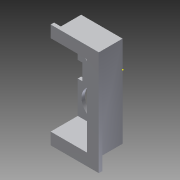
# Autodesk Inventor part: Sonar_Bracket
Saved by Autodesk Inventor 2015 (Build 190159000, 159)
## iProperties
Created: 2017-03-19
Part Number: Sonar_Bracket
Material: ABS Plastic
Document SubType Name: Modeling
Designer: ks2101
Density: 1.06 g/cm^3
Appearance: Smooth - White
Author: ks2101
Autodesk Inventor part; units mm, degrees
ref_plane "YZ Plane" through (0, 0, 0) normal (1, 0, 0) x (0, 1, 0)
ref_plane "XZ Plane" through (0, 0, 0) normal (0, 1, 0) x (-1, 0, 0)
ref_plane "XY Plane" through (0, 0, 0) normal (0, 0, 1) x (1, 0, 0)
sketch "Sketch1" plane through (0, 0, 0) normal (0, 0, 1) x (1, 0, 0)
  line L0 (-2.6984, 15.8681) -> (21.7216, 15.8681)
  line L1 (21.7216, 15.8681) -> (21.7216, -37.8319)
  line L2 (21.7216, -37.8319) -> (-2.6984, -37.8319)
  line L3 (-2.6984, -37.8319) -> (-2.6984, 15.8681)
  point P0 (0, 0)
  dimension "d0" = 53.7
  dimension "d1" = 24.42
  constraints: 8 end point, 2 parallel, 1 horizontal, 1 perpendicular
  measures "d0" distance of L1.end L0.end
  measures "d1" distance of L0.start L0.end
extrude "Extrusion1" add sketch "Sketch1" along normal blind 2
sketch "Sketch2" plane through (0, 0, 2) normal (0, 0, 1) x (1, 0, 0)
  line L0 (-2.6984, -37.8319) -> (21.7216, -37.8319) projected
  line L1 (21.7216, 15.8681) -> (18.7216, 15.8681)
  line L2 (18.7216, 15.8681) -> (18.7216, -37.8319)
  line L3 (18.7216, -37.8319) -> (21.7216, -37.8319)
  line L4 (21.7216, -37.8319) -> (21.7216, 15.8681)
  line L5 (21.7216, -37.8319) -> (21.7216, 15.8681) projected
  line L6 (-2.6984, 15.8681) -> (21.7216, 15.8681)
  line L7 (21.7216, 15.8681) -> (21.7216, 12.8681)
  line L8 (21.7216, 12.8681) -> (-2.6984, 12.8681)
  line L9 (-2.6984, 12.8681) -> (-2.6984, 15.8681)
  line L10 (-2.6984, -37.8319) -> (21.7216, -37.8319)
  line L11 (21.7216, -37.8319) -> (21.7216, -34.8319)
  line L12 (21.7216, -34.8319) -> (-2.6984, -34.8319)
  line L13 (-2.6984, -34.8319) -> (-2.6984, -37.8319)
  point P0 (0, 0)
  dimension "d4" = 3
  dimension "d5" = 3
  dimension "d6" = 3
  constraints: 24 end point, 6 parallel, 3 horizontal, 3 perpendicular, 3 point on line
  measures "d4" distance of L1.start L1.end
  measures "d5" distance of L7.end L6.end
  measures "d6" distance of L0.end L11.end
extrude "Extrusion2" add sketch "Sketch2" along normal blind 16
sketch "Sketch3" plane through (0, 0, 0) normal (0, 0, -1) x (-1, 0, 0)
  point P0 (0, 0)
sketch "Sketch4" plane through (0, 0, 0) normal (0, 0, -1) x (-1, 0, 0)
  circle A0 centre (-8.0116, 2.4017) radius 8.5
  circle A1 centre (-8.0116, -24.3699) radius 8.5
  line L0 (2.6984, -37.8319) -> (2.6984, 15.8681) projected
  line L1 (-21.7216, -37.8319) -> (2.6984, -37.8319) projected
  line L2 (2.6984, 15.8681) -> (-21.7216, 15.8681) projected
  line L3 (-18.7216, 12.8681) -> (-18.7216, -34.8319) projected
  point P0 (0, 0)
  dimension "d9" = 17
  dimension "d10" = 17
  dimension "d11" = 10.71
  dimension "d12" = 10.71
  dimension "d13" = 26.7716
  dimension "d14" = 13.462
  dimension "d15" = 13.4664
  dimension "d45" = 24.42
  dimension "d46" = 21.42
  constraints: 2 centre point
  measures "d9" diameter of A0
  measures "d10" diameter of A1
  measures "d11" distance from line of L0 A0.centre
  measures "d12" distance from line of L0 A1.centre
  measures "d13" distance of A1.centre A0.centre
  measures "d14" distance from line of L1 A1.centre
  measures "d15" distance from line of L2 A0.centre
  measures "d45" distance of L0.end L2.end
  measures "d46" distance between parallel lines of L3 L0
hole "Hole1" at (8.0116, 2.4017, 0) at (8.0116, -24.3699, 0) direction (0, 0, 1) diameter 17 depth 2 tip angle 118
sketch "Sketch5" plane through (0, 0, 2) normal (0, 0, 1) x (1, 0, 0)
  line L0 (-0.1076, -6.2299) -> (-2.6984, -6.2299)
  line L1 (-2.6984, -6.2299) -> (-2.6984, -15.7299)
  line L2 (-2.6984, -15.7299) -> (-0.1076, -15.7299)
  line L3 (-0.1076, -15.7299) -> (-0.1076, -6.2299)
  line L4 (21.7216, 15.8681) -> (-2.6984, 15.8681) projected
  line L5 (-2.6984, -37.8319) -> (21.7216, -37.8319) projected
  line L6 (-2.6984, 12.8681) -> (-2.6984, -34.8319) projected
  point P0 (0, 0)
  dimension "d23" = 9.5
  dimension "d24" = 22.098
  dimension "d25" = 22.102
  dimension "d26" = 2.5908
  dimension "d27" = 0
  dimension "d47" = 2.5908
  constraints: 8 end point, 2 parallel, 1 horizontal, 1 perpendicular
  measures "d23" distance of L0.end L1.end
  measures "d24" distance from line of L0.start L4
  measures "d25" distance between parallel lines of L2 L5
  measures "d26" distance of L1.end L2.end
  measures "d27" distance between parallel lines of L6 L1
  measures "d47" distance between parallel lines of L3 L6
extrude "Extrusion3" cut sketch "Sketch5" against normal blind 10
sketch "Sketch6" plane through (0, 0, 2) normal (0, 0, 1) x (1, 0, 0)
  line L0 (17.7216, -5.7319) -> (13.7216, -5.7319)
  line L1 (13.7216, -5.7319) -> (13.7216, -16.2319)
  line L2 (13.7216, -16.2319) -> (17.7216, -16.2319)
  line L3 (17.7216, -16.2319) -> (17.7216, -5.7319)
  line L4 (21.7216, 15.8681) -> (21.7216, -37.8319) projected
  line L5 (-2.6984, -37.8319) -> (21.7216, -37.8319) projected
  line L6 (21.7216, 15.8681) -> (-2.6984, 15.8681) projected
  point P0 (0, 0)
  dimension "d30" = 4
  dimension "d31" = 10.5
  dimension "d32" = 4
  dimension "d33" = 21.6
  dimension "d34" = 21.6
  constraints: 8 end point, 2 parallel, 1 horizontal, 1 perpendicular
  measures "d30" distance of L0.start L0.end
  measures "d31" distance of L0.end L1.end
  measures "d32" distance between parallel lines of L4 L3
  measures "d33" distance between parallel lines of L5 L2
  measures "d34" distance between parallel lines of L6 L0
extrude "Extrusion4" cut sketch "Sketch6" against normal blind 10
sketch "Sketch7" plane through (-2.6984, 15.8681, 0) normal (0, 1, 0) x (1, 0, 0)
  line L0 (0, -2) -> (0, -18) projected
  line L1 (24.42, -18) -> (0, -18)
  line L2 (0, -18) -> (0, -16)
  line L3 (0, -16) -> (24.42, -16)
  line L4 (24.42, -16) -> (24.42, -18)
  point P0 (2.6984, 0)
  dimension "d37" = 2
  constraints: 8 end point, 2 parallel, 1 horizontal, 1 perpendicular, 1 point on line
  measures "d37" distance of L2.end L0.end
extrude "Extrusion5" add sketch "Sketch7" along normal blind 4
sketch "Sketch8" plane through (21.7216, -37.8319, 0) normal (1, 0, 0) x (0, 0, -1)
  point P0 (0, 37.8319)
sketch "Sketch9" plane through (-2.6984, -37.8319, 0) normal (0, -1, 0) x (1, 0, 0)
  line L0 (24.42, 0) -> (24.42, 18) projected
  line L1 (0, 18) -> (24.42, 18)
  line L2 (24.42, 18) -> (24.42, 16)
  line L3 (24.42, 16) -> (0, 16)
  line L4 (0, 16) -> (0, 18)
  point P0 (2.6984, 0)
  dimension "d40" = 2
  constraints: 8 end point, 2 parallel, 1 horizontal, 1 perpendicular, 1 point on line
  measures "d40" distance of L3.end L1.start
extrude "Extrusion6" add sketch "Sketch9" along normal blind 4
sketch "Sketch10" plane through (21.7216, -37.8319, 0) normal (1, 0, 0) x (0, 0, -1)
  line L0 (-18, -4) -> (-16, -4)
  line L1 (-16, -4) -> (-16, 57.7)
  line L2 (-16, 57.7) -> (-18, 57.7)
  line L3 (-18, 57.7) -> (-18, -4)
  point P0 (0, 37.8319)
  constraints: 8 end point, 2 parallel, 1 horizontal, 1 perpendicular
extrude "Extrusion7" add sketch "Sketch10" along normal blind 4
equation "\"d11\" = 0.5 * d46"
equation "\"d12\" = 0.5 * d46"
equation "\"d33\" = d34"
body "Solid1"
